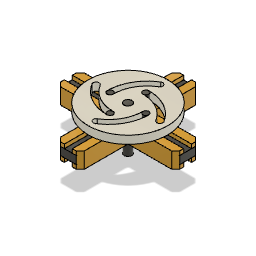
slot_cam_four_sliding (Autodesk Fusion 360 design; units mm, degrees)
Autodesk Fusion 360 part; units mm, degrees
sketch "Sketch1" plane through (0, 0, 0) normal (0, 1, 0) x (1, 0, 0)
  circle A0 centre (0, 0) radius 50
  line L0 (0, 0) -> (0, 22.5) construction
  line L1 (0, 0) -> (40, 0) construction
  arc A1 (43.2047, 1.9473) -> (0, 26.25) centre (0, -24.3056) ccw
  arc A2 (36.7953, -1.9473) -> (43.2047, 1.9473) centre (40, 0) ccw
  arc A3 (36.7953, -1.9473) -> (0, 18.75) centre (0, -24.3056) ccw
  arc A4 (0, 26.25) -> (0, 18.75) centre (0, 22.5) ccw
  arc A5 (40, 0) -> (0, 22.5) centre (0, -24.3056) ccw construction
  line L2 (0, 22.5) -> (50.2081, 22.5) construction
  line L3 (40, 0) -> (40, 22.5) construction
  arc A6 (1.9473, 36.7953) -> (-18.75, 0) centre (24.3056, 0) ccw
  arc A7 (1.9473, 36.7953) -> (-1.9473, 43.2047) centre (0, 40) ccw
  arc A8 (-1.9473, 43.2047) -> (-26.25, 0) centre (24.3056, 0) ccw
  arc A9 (-26.25, 0) -> (-18.75, 0) centre (-22.5, 0) ccw
  arc A10 (-36.7953, 1.9473) -> (0, -18.75) centre (0, 24.3056) ccw
  arc A11 (-36.7953, 1.9473) -> (-43.2047, -1.9473) centre (-40, 0) ccw
  arc A12 (-43.2047, -1.9473) -> (0, -26.25) centre (0, 24.3056) ccw
  arc A13 (0, -26.25) -> (0, -18.75) centre (0, -22.5) ccw
  arc A14 (-1.9473, -36.7953) -> (18.75, 0) centre (-24.3056, 0) ccw
  arc A15 (-1.9473, -36.7953) -> (1.9473, -43.2047) centre (0, -40) ccw
  arc A16 (1.9473, -43.2047) -> (26.25, 0) centre (-24.3056, 0) ccw
  arc A17 (26.25, 0) -> (18.75, 0) centre (22.5, 0) ccw
  circle A18 centre (0, 0) radius 5
  dimension "d1" = 100
  dimension "d2" = 22.5
  dimension "d3" = 40
  dimension "d4" = 7.5
  dimension "d6" = 360
  dimension "d7" = 10
  constraint coincident A0.centre L0.start
  constraint vertical L0
  constraint perpendicular L0 L1
  constraint tangent A1 A2
  constraint tangent A2 A3
  constraint tangent A3 A4
  constraint tangent A1 A4
  constraint coincident L1.end A2.centre
  constraint coincident L0.end A4.centre
  constraint horizontal L2
  constraint tangent A5 L2
  constraint coincident L2 L3.end
  constraint perpendicular L2 L3
  measures "d1" diameter of A0 L0.start
  measures "d2" distance of A0.centre L0.end
  measures "d3" distance of A0.centre L1.end
  measures "d4" diameter of A4
  measures "d7" diameter of A18
  measures "d28" distance of A0.centre
extrude "Extrude1" add sketch "Sketch1" along normal blind 10 makes body 1 in component "Component"
sketch "Sketch1 (2)" plane through (0, 0, 0) normal (0, 1, 0) x (1, 0, 0) in component "Component'"
  circle A0 centre (0, 0) radius 50
  line L0 (75, -15) -> (-75, -15)
  line L1 (-75, -15) -> (-75, 15)
  line L2 (-75, 15) -> (75, 15)
  line L3 (75, 15) -> (75, -15)
  line L4 (75, -15) -> (-75, 15) construction
  line L5 (-75, -15) -> (75, 15) construction
  line L6 (75, -5) -> (-75, -5)
  line L7 (-75, -5) -> (-75, 5)
  line L8 (-75, 5) -> (75, 5)
  line L9 (75, 5) -> (75, -5)
  line L10 (75, -5) -> (-75, 5) construction
  line L11 (-75, -5) -> (75, 5) construction
  line L12 (0, 15) -> (0, -15)
  line L13 (0, 15) -> (5, 15)
  line L14 (5, 15) -> (5, -15)
  line L15 (5, -15) -> (0, -15)
  line L16 (0, -15) -> (0, 15)
  dimension "d10" = 150
  dimension "d11" = 30
  dimension "d12" = 10
  dimension "d20" = 5
  constraint perpendicular L0 L1
  constraint parallel L0 L2
  constraint parallel L1 L3
  constraint horizontal L0
  constraint coincident L4 A0.centre
  constraint coincident L5 A0.centre
  constraint coincident A0.centre origin
  constraint perpendicular L6 L7
  constraint parallel L6 L8
  constraint parallel L7 L9
  constraint horizontal L6
  constraint coincident L10 A0.centre
  constraint coincident L11 A0.centre
  constraint midpoint L2 L12.start
  constraint midpoint L0 L12.end
  constraint horizontal L13
  constraint vertical L14
  constraint horizontal L15
  constraint vertical L16
  measures "d10" distance of L1.end L2.end
  measures "d11" distance of L0.end L1.end
  measures "d12" distance of L6.end L7.end
  measures "d20" distance of L12.start L13.end
extrude "Extrude1'" add sketch "Sketch1 (2)" against normal blind 20 separate body contours A0 L2 L8 L14 | A0 L2 L3 L8 | A0 L0 L3 L6 | A0 L0 L6 L14 makes body 2 at (28.3333, -6.6667, -5) makes body 3 at (51.6667, -6.6667, 5) in component "Component'"
sketch "Sketch2" plane through (75, 0, 0) normal (1, 0, 0) x (0, 0, -1) in component "Component'"
  line L0 (-5, 0) -> (-15, 0)
  line L1 (-15, 0) -> (-15, -20)
  line L2 (-15, -20) -> (-5, -20)
  line L3 (-5, -20) -> (-5, 0)
  line L4 (-10, -5) -> (10, -5)
  line L5 (10, -5) -> (10, -15)
  line L6 (10, -15) -> (-10, -15)
  line L7 (-10, -15) -> (-10, -5)
  dimension "d15" = 20
  dimension "d16" = 5
  dimension "d17" = 5
  dimension "d27" = 10
  constraint horizontal L4
  constraint vertical L5
  constraint horizontal L6
  constraint vertical L7
  measures "d15" distance of L4.start L4.end
  measures "d16" distance of L1 L7
  measures "d17" distance of L2 L6
  measures "d27" distance of L4.start L6.end
extrude "Extrude2" cut sketch "Sketch2" against normal blind 240 contours L3 L4 L5 L6 | L3 L4 L6 L7 bodies 2 3 in component "Component'"
chamfer "Chamfer1" distance 5 angle 45 2 edges at (75, -10, 15) (75, -10, -15) on bodies 2 3 in component "Component'"
pattern_circular "C-Pattern1" count 4 over 360 about axis through (0, 1.75, 0) along (0, 1, 0) of bodies 2 3 makes body 4 at (15, -13.3333, -48.3334) makes body 5 at (-48.3334, -13.3333, -15) makes body 6 at (-15, -13.3333, 48.3334) makes body 7 at (-15, -6.6667, -26.667) makes body 8 at (-26.667, -6.6667, 15) makes body 9 at (15, -13.3333, 26.667) in component "Component'"
sketch "Sketch1 (3)" plane through (0, 0, 75) normal (0, 0, 1) x (1, 0, 0) in component "Component''"
  line L0 (-10, 0) -> (-10, -5)
  line L1 (-10, -5) -> (-5, -5)
  line L2 (-5, -5) -> (-5, 0)
  line L3 (-5, 0) -> (-10, 0)
  line L4 (-10, -5) -> (10, -5)
  line L5 (10, -5) -> (10, -15)
  line L6 (10, -15) -> (-10, -15)
  line L7 (-10, -15) -> (-10, -5)
  line L8 (-5, -20) -> (-10, -20)
  dimension "d24" = 20
  dimension "d26" = 5
  dimension "d28" = 10
  constraint horizontal L4
  constraint vertical L5
  constraint horizontal L6
  constraint vertical L7
  constraint coincident L0.end L1.start
  measures "d24" distance of L0.end L4.end
  measures "d26" distance of L6 L8
  measures "d28" distance of L0.end L6.end
extrude "Extrude1''" add sketch "Sketch1 (3)" against normal blind 60 separate body contours L1 L4 L5 L6 L7 makes body 10 in component "Component''"
sketch "Sketch2 (2)" plane through (0, -5, 0) normal (0, 1, 0) x (-1, 0, 0) in component "Component''"
  line L0 (10, 75) -> (-10, 75)
  line L1 (-10, 75) -> (-10, 15)
  line L2 (-10, 15) -> (10, 15)
  line L3 (10, 15) -> (10, 75)
  arc A0 (1.9473, 36.7953) -> (-1.9473, 43.2047) centre (0, 40) ccw
  arc A1 (0, 26.25) -> (0, 18.75) centre (0, 22.5) ccw
  circle A2 centre (0, 22.5) radius 3.75
  constraint concentric A1 A2
  constraint coincident A1.start A2
extrude "Extrude2'" add sketch "Sketch2 (2)" along normal blind 15 contours A1 A2 bodies 10 in component "Component''"
pattern_circular "C-Pattern1'" count 4 over 360 about axis through (0, 1.75, 0) along (0, 1, 0) of bodies 10 makes body 11 at (35, -15, -3.3333) makes body 12 at (-3.3333, -15, -55) makes body 13 at (-35, -15, 3.3333) in component "Component''"
copy_body "Body->Comp1" bodies 10 removing the originals makes body 14 in component "Component'''"
copy_body "Body->Comp2" bodies 11 removing the originals makes body 15 in component "Component''''"
copy_body "Body->Comp3" bodies 12 removing the originals makes body 16 in component "Component'''''"
copy_body "Body->Comp4" bodies 13 removing the originals makes body 17 in component "Component''''''"
combine "Combine1" operation add target body 6 tool bodies 8 in component "Component'"
combine "Combine2" operation add target body 9 tool bodies 3 in component "Component'"
combine "Combine3" operation add target body 5 tool bodies 7 in component "Component'"
combine "Combine4" operation add target body 2 tool bodies 4 in component "Component'"
cylinder "CylinderPrimitive1" add diameter 10 height -55 placed x (1, 0, 0) y (0, 0, -1) z (0, 1, 0) at (0, 10, 0) separate body makes body 18 in component "Component'''''''"
component "Component" placed x (1, 0, 0) y (0, 1, 0) z (0, 0, 1) at (0, 0, 0)
component "Component'" placed x (1, 0, 0) y (0, 1, 0) z (0, 0, 1) at (0, 0, 0)
component "Component''" placed x (1, 0, 0) y (0, 1, 0) z (0, 0, 1) at (0, 0, 0)
component "Component'''''''" placed x (1, 0, 0) y (0, 1, 0) z (0, 0, 1) at (0, 0, 0)
component "Component'''" placed x (1, 0, 0) y (0, 1, 0) z (0, 0, 1) at (0, 0, 0) in component "Component''"
component "Component''''" placed x (1, 0, 0) y (0, 1, 0) z (0, 0, 1) at (0, 0, 0) in component "Component''"
component "Component'''''" placed x (1, 0, 0) y (0, 1, 0) z (0, 0, 1) at (0, 0, 0) in component "Component''"
component "Component''''''" placed x (1, 0, 0) y (0, 1, 0) z (0, 0, 1) at (0, 0, 0) in component "Component''"
